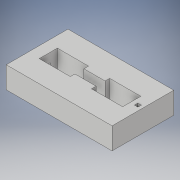
# Autodesk Inventor part: ODS_Enclosure_Mid_V2D4
Saved by Autodesk Inventor 2017 (Build 210142000, 142)
## iProperties
Created: 2017-12-28
Part Number: ODS_Enclosure_Mid_V2D4
Material: Generic
Document SubType Name: Modeling
Designer: Tripl_000
Density: 1 g/cm^3
Appearance: Default
Author: Tripl_000
Autodesk Inventor part; units mm, degrees
ref_plane "YZ Plane" through (0, 0, 0) normal (1, 0, 0) x (0, 1, 0)
ref_plane "XZ Plane" through (0, 0, 0) normal (0, 1, 0) x (-1, 0, 0)
ref_plane "XY Plane" through (0, 0, 0) normal (0, 0, 1) x (1, 0, 0)
sketch "Sketch1" plane through (0, 0, 0) normal (0, 1, 0) x (-1, 0, 0)
  line L0 (76.2, 44.45) -> (-76.2, 44.45)
  line L1 (-76.2, 44.45) -> (-76.2, -44.45)
  line L2 (-76.2, -44.45) -> (76.2, -44.45)
  line L3 (76.2, -44.45) -> (76.2, 44.45)
  line L4 (76.2, 44.45) -> (-76.2, -44.45) construction
  line L5 (-76.2, 44.45) -> (76.2, -44.45) construction
  point P0 (0, 0)
  dimension "d0" = 152.4
  dimension "d1" = 88.9
  constraints: 12 end point, 2 midpoint, 2 parallel, 1 horizontal, 1 perpendicular
  measures "d0" distance of L1.end L2.end
  measures "d1" distance of L2.end L0.start
extrude "Extrusion1" add sketch "Sketch1" along normal blind 31.242
sketch "Sketch2" plane through (0, 31.242, 0) normal (0, 1, 0) x (1, 0, 0)
  line L0 (-60.071, -13.081) -> (60.071, -13.081)
  line L1 (60.071, -13.081) -> (60.071, 13.081)
  line L2 (60.071, 13.081) -> (-60.071, 13.081)
  line L3 (-60.071, 13.081) -> (-60.071, -13.081)
  line L4 (-60.071, -13.081) -> (60.071, 13.081) construction
  line L5 (60.071, -13.081) -> (-60.071, 13.081) construction
  point P0 (0, 0)
  dimension "d4" = 120.142
  dimension "d5" = 26.162
  constraints: 12 end point, 2 midpoint, 2 parallel, 1 horizontal, 1 perpendicular
  measures "d4" distance of L1.end L2.end
  measures "d5" distance of L2.end L0.start
extrude "Extrusion2" cut sketch "Sketch2" against normal through all
ref_plane "Work Plane1" through (-76.2, 0, 0) normal (0, 0, 1) x (1, 0, 0)
sketch "Sketch4" plane through (-60.071, 31.242, -13.081) normal (0, 0, 1) x (1, 0, 0)
  line L0 (0, 0) -> (120.142, 0) projected
  line L1 (120.142, -31.242) -> (0, -31.242) projected
  line L2 (44.831, 0) -> (75.311, 0)
  line L3 (75.311, 0) -> (75.311, -31.242)
  line L4 (75.311, -31.242) -> (44.831, -31.242)
  line L5 (44.831, -31.242) -> (44.831, 0)
  line L6 (120.142, 0) -> (120.142, -31.242) projected
  point P0 (60.071, -31.242)
  dimension "d13" = 30.48
  dimension "d14" = 44.831
  constraints: 8 end point, 2 parallel, 2 point on line, 1 horizontal, 1 perpendicular
  measures "d13" distance between parallel lines of L3 L5
  measures "d14" distance between parallel lines of L6 L3
extrude "Extrusion3" add sketch "Sketch4" along normal blind 6.6548 contours L0 L3 L1 L5
mirror "Mirror1" about plane through (-76.2, 0, 0) normal (0, 0, 1) of "Extrusion3"
ref_plane "Work Plane2" through (0, 0, 44.45) normal (1, 0, 0) x (0, 0, -1)
sketch "Sketch6" plane through (-60.071, 31.242, 13.081) normal (1, 0, 0) x (0, 0, -1)
  line L0 (15.621, -13.081) -> (10.541, -13.081)
  line L1 (10.541, -13.081) -> (10.541, -18.161)
  line L2 (10.541, -18.161) -> (15.621, -18.161)
  line L3 (15.621, -18.161) -> (15.621, -13.081)
  line L4 (15.621, -13.081) -> (10.541, -18.161) construction
  line L5 (10.541, -13.081) -> (15.621, -18.161) construction
  line L6 (26.162, 0) -> (26.162, -31.242) projected
  point P0 (13.081, -31.242)
  point P1 (13.081, -15.621)
  dimension "d31" = 15.621
  dimension "d32" = 13.081
  dimension "d33" = 5.08
  dimension "d34" = 5.08
  constraints: 12 end point, 2 midpoint, 2 parallel, 1 horizontal, 1 perpendicular
  measures "d31" distance of point (13.081, -31.242) point (13.081, -15.621)
  measures "d32" distance from line of L6 point (13.081, -15.621)
  measures "d33" distance of L2.end L0.start
  measures "d34" distance of L1.end L2.end
extrude "Extrusion5" cut sketch "Sketch6" against normal blind 11.43
mirror "Mirror2" about plane through (0, 0, 44.45) normal (1, 0, 0) of "Extrusion5"
sketch "Sketch7" plane through (0, 31.242, 0) normal (0, 1, 0) x (1, 0, 0)
  line L0 (71.501, -2.54) -> (71.501, 2.54) projected
  line L1 (60.071, 2.54) -> (71.501, 2.54) projected
  line L2 (71.501, -2.54) -> (66.421, -2.54)
  line L3 (66.421, -2.54) -> (66.421, 2.54)
  line L4 (66.421, 2.54) -> (71.501, 2.54)
  line L5 (71.501, 2.54) -> (71.501, -2.54)
  point P0 (0, 0)
  dimension "d37" = 5.08
  constraints: 8 end point, 2 parallel, 1 horizontal, 1 perpendicular, 1 point on line
  measures "d37" distance between parallel lines of L0 L3
extrude "Extrusion6" cut sketch "Sketch7" against normal up to next
sketch "Sketch8" plane through (0, 0, 0) normal (0, -1, 0) x (1, 0, 0)
  line L0 (-71.501, 2.54) -> (-71.501, -2.54) projected
  line L1 (-60.071, -2.54) -> (-71.501, -2.54) projected
  line L2 (-71.501, 2.54) -> (-66.4254, 2.54)
  line L3 (-66.4254, 2.54) -> (-66.4254, -2.54)
  line L4 (-66.4254, -2.54) -> (-71.501, -2.54)
  line L5 (-71.501, -2.54) -> (-71.501, 2.54)
  point P0 (0, 0)
  constraints: 8 end point, 2 parallel, 1 horizontal, 1 perpendicular, 1 point on line
extrude "Extrusion7" cut sketch "Sketch8" against normal up to next
fillet "Fillet1" radius 3.175 1 edges at (-71.501, 18.161, 0)
fillet "Fillet2" radius 3.175 1 edges at (66.421, 18.161, 0)
fillet "Fillet3" radius 3.175 1 edges at (-66.4254, 13.081, 0)
fillet "Fillet4" radius 3.175 1 edges at (71.501, 13.081, 0)
body "Solid1"
